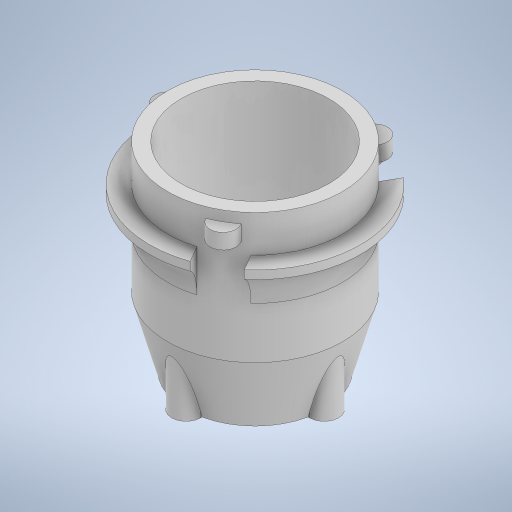
# Autodesk Inventor part: Diffuser Nozzle
Saved by Autodesk Inventor 2023.2 (Build 272271000, 271)
## iProperties
Created: 2024-07-24
Part Number: Diffuser Nozzle
Material: Типовые
Document SubType Name: Modeling
Designer: user
Density: 1 g/cm^3
Appearance: По умолчанию
Author: user
Autodesk Inventor part; units mm, degrees
ref_plane "YZ Plane" through (0, 0, 0) normal (1, 0, 0) x (0, 1, 0)
ref_plane "XZ Plane" through (0, 0, 0) normal (0, 1, 0) x (-1, 0, 0)
ref_plane "XY Plane" through (0, 0, 0) normal (0, 0, 1) x (1, 0, 0)
sketch "Эскиз1" plane through (0, 0, 0) normal (0, 1, 0) x (-1, 0, 0)
  circle A0 centre (0, 0) radius 13.05
  circle A1 centre (0, 0) radius 15.45
  dimension "d0" = 26.1
  dimension "d1" = 30.9
  constraints: 2 centre point, 2 coincident
  measures "d0" diameter of A0
  measures "d1" diameter of A1
extrude "Выдавливание1" add sketch "Эскиз1" against normal blind 19.5
sketch "Эскиз2" plane through (0, -19.5, 0) normal (0, -1, 0) x (1, 0, 0)
  point P0 (0, 0)
sketch "Эскиз3" plane through (0, 0, 0) normal (0, 0, 1) x (1, 0, 0)
  line L0 (-15.45, -19.5) -> (15.45, -19.5) projected
  line L1 (0, -19.5) -> (-12.25, -19.5)
  line L2 (0, -19.5) -> (0, -31.5)
  line L3 (0, -31.5) -> (-10.85, -31.5)
  line L4 (-12.25, -19.5) -> (-10.85, -31.5)
  line L5 (0, -19.5) -> (-15.45, -19.5)
  line L6 (0, -31.5) -> (-12.2, -31.5)
  line L7 (-15.45, -19.5) -> (-12.2, -31.5)
  point P0 (0, 0)
  dimension "d5" = 12.25
  dimension "d6" = 12
  dimension "d7" = 10.85
  dimension "d8" = 12.2
  constraints: 14 end point, 1 collinear, 1 midpoint, 1 parallel, 1 perpendicular, 1 point on line
  measures "d5" distance of L1.start L1.end
  measures "d6" distance of L1.start L2.end
  measures "d7" distance of L2.end L3.end
  measures "d8" distance of L2.end L6.end
revolve "Вращение1" add sketch "Эскиз3" angle 360 about axis through (0, -19.5, 0) along (0, -1, 0) contours L0 L4 L6 L7
sketch "Эскиз4" plane through (0, -31.5, 0) normal (0, -1, 0) x (1, 0, 0)
  circle A0 centre (0, 0) radius 12.2 projected
  arc A1 (-2.55, -12.2) -> (2.55, -12.2) centre (0, -12.2) ccw
  line L0 (0, -12.2) -> (2.55, -12.2)
  line L1 (2.55, -12.2) -> (2.55, -11.9305)
  line L2 (0, -12.2) -> (-2.55, -12.2)
  line L3 (-2.55, -12.2) -> (-2.55, -11.9305)
  line L4 (2.55, -11.9305) -> (-2.55, -11.9305)
  point P0 (0, 0)
  dimension "d10" = 5.1
  constraints: 10 end point, 5 point on circle, 2 perpendicular, 1 centre point, 1 horizontal, 1 tangent, 1 vertical
  measures "d10" diameter of A1
extrude "Выдавливание2" add sketch "Эскиз4" against normal through all contours A0 L2 L3 | L1 L0 A0 | L0 A1 L2
pattern_circular "Круговой массив1" count 4 over 360 about axis through (0, -10, 0) along (0, 1, 0) of "Выдавливание2"
extrude "Выдавливание3" add sketch "Эскиз1" along normal blind 3.5
sketch "Эскиз5" plane through (0, 3.5, 0) normal (0, 1, 0) x (1, 0, 0)
  circle A0 centre (0, 0) radius 18.625
  circle A1 centre (0, 0) radius 15.45
  line L0 (-18.625, 0) -> (-18.625, -3.5)
  line L1 (-18.625, -3.5) -> (-15.0483, -3.5)
  circle A2 centre (0, 0) radius 15.45 projected
  line L2 (-18.625, 0) -> (-15.45, 0)
  line L3 (-18.625, 0) -> (-18.625, 3.5)
  line L4 (-18.625, 3.5) -> (-15.0483, 3.5)
  line L5 (9.3125, 16.1297) -> (6.2814, 17.8797)
  line L6 (6.2814, 17.8797) -> (4.4931, 14.7822)
  line L7 (9.3125, 16.1297) -> (12.3436, 14.3797)
  line L8 (12.3436, 14.3797) -> (10.5553, 11.2822)
  line L9 (9.3125, -16.1297) -> (12.3436, -14.3797)
  line L10 (12.3436, -14.3797) -> (10.5553, -11.2822)
  line L11 (9.3125, -16.1297) -> (6.2814, -17.8797)
  line L12 (6.2814, -17.8797) -> (4.4931, -14.7822)
  point P0 (12.1777, -14.0924)
  point P1 (12.1777, 14.0924)
  point P2 (6.1155, -17.5924)
  point P3 (-18.2932, -3.5)
  point P4 (6.1155, 17.5924)
  point P5 (-18.2932, 3.5)
  dimension "d18" = 37.25
  dimension "d19" = 3.5
  dimension "d22" = 360
  constraints: 26 end point, 4 coincident, 2 point on circle, 2 symmetric about line, 2 vertical, 1 centre point, 1 horizontal, 1 perpendicular, 32 other
  measures "d19" distance of L0.start L0.end
extrude "Выдавливание4" add sketch "Эскиз5" against normal blind 8.05 contours A0 L10 A1 L8 | L6 A1 L4 A0 | A0 L1 A1 L12
extrude "Выдавливание5" cut sketch "Эскиз5" against normal blind 6.55 contours A0 L10 A1 L8 | L6 A1 L4 A0 | A0 L1 A1 L12
fillet "Сопряжение1" radius 7 3 edges at (-7.725, -4.55, 13.3801) (-7.725, -4.55, -13.3801) (15.45, -4.55, 0)
sketch "Эскиз6" plane through (0, 3.5, 0) normal (0, 1, 0) x (1, 0, 0)
  line L0 (12.1777, -14.0924) -> (6.1155, -17.5924)
  line L1 (9.1466, -15.8424) -> (7.725, -13.3801)
  circle A0 centre (0, 0) radius 15.45 projected
  line L2 (7.725, -13.3801) -> (8.725, -15.1121)
  circle A1 centre (7.725, -13.3801) radius 2.3
  point P0 (9.6257, -12.085)
  point P1 (5.6531, -14.3786)
  dimension "d29" = 2
  dimension "d30" = 4.6
  constraints: 6 end point, 1 centre point, 1 coincident, 1 midpoint, 1 point on line, 2 other
  measures "d29" distance of L1.end L2.end
  measures "d30" diameter of A1
extrude "Выдавливание6" add sketch "Эскиз6" against normal blind 4.5 contours L1 A1 A0 | L1 A0 A1 | A0 A1 picked at (6.965, -12.9536)
extrude "Выдавливание7" cut sketch "Эскиз6" against normal blind 1.8 contours L1 A1 A0 | L1 A0 A1
pattern_circular "Круговой массив2" count 3 over 360 about axis through (0, -10, 0) along (0, 1, 0) of "Выдавливание6", "Выдавливание7"
